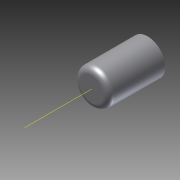
# Autodesk Inventor part: GearBoxPin
Saved by Autodesk Inventor 2012 (Build 160160000, 160)
## iProperties
Created: 2011-12-02
Part Number: GearBoxPin
Material: Default
Document SubType Name: Modeling
Designer: Drew
Density: 1 g/cm^3
Author: Drew
Autodesk Inventor part; units mm, degrees
ref_plane "YZ Plane" through (0, 0, 0) normal (1, 0, 0) x (0, 1, 0)
ref_plane "XZ Plane" through (0, 0, 0) normal (0, 1, 0) x (-1, 0, 0)
ref_plane "XY Plane" through (0, 0, 0) normal (0, 0, 1) x (1, 0, 0)
sketch "Sketch1" plane through (0, 0, 0) normal (0, 0, 1) x (1, 0, 0)
  circle A0 centre (0, 0) radius 1.5
  dimension "d0" = 3
  constraints: 1 centre point, 1 coincident
  measures "d0" diameter of A0
extrude "Extrusion1" add sketch "Sketch1" along normal blind 4.8
fillet "Fillet1" radius 0.5 1 edges at (-1.5, 0, 4.8)
body "Solid1"
